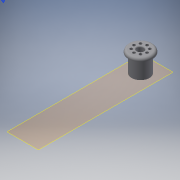
# Autodesk Inventor part: qsd
Saved by Autodesk Inventor 2018 (Build 220112000, 112)
## iProperties
Created: 2019-11-22
Part Number: qsd
Material: Generic
Document SubType Name: Modeling
Designer: bitbots
Density: 1 g/cm^3
Appearance: Default
Author: bitbots
Autodesk Inventor part; units mm, degrees
ref_plane "YZ Plane" through (0, 0, 0) normal (1, 0, 0) x (0, 1, 0)
ref_plane "XZ Plane" through (0, 0, 0) normal (0, 1, 0) x (-1, 0, 0)
ref_plane "XY Plane" through (0, 0, 0) normal (0, 0, 1) x (1, 0, 0)
ref_plane "Work Plane1" through (0, 0, 0) normal (0, 0, 1) x (1, 0, 0)
sketch "Sketch1" plane through (0, 0, 0) normal (0, 0, 1) x (1, 0, 0)
  line L0 (-11.048, 15.3384) -> (-24.0178, 163.5839) projected
  arc A0 (-11.7363, 13.6476) -> (-11.048, 15.3384) centre (-13.0404, 15.1641) ccw projected
  arc A1 (-11.7363, 13.6476) -> (9, -15.5885) centre (0, 0) ccw projected
  line L1 (13.9461, -12.7329) -> (9, -15.5885) projected
  arc A2 (13.9461, -12.7329) -> (23.8699, 6.3308) centre (3.9461, 4.5877) ccw projected
  line L2 (10.9035, 154.5385) -> (23.8699, 6.3308) projected
  arc A3 (11.6063, 156.2416) -> (10.9035, 154.5385) centre (12.8958, 154.7128) ccw projected
  arc A4 (11.6063, 156.2416) -> (-9, 185.5885) centre (0, 170) ccw projected
  line L3 (-14.0939, 182.6475) -> (-9, 185.5885) projected
  arc A5 (-14.0939, 182.6475) -> (-24.0178, 163.5839) centre (-4.0939, 165.327) ccw projected
  circle A6 centre (0, 0) radius 5.5 projected
  circle A7 centre (0, 170) radius 5.5 projected
  circle A8 centre (0, -11) radius 1.35 projected
  circle A9 centre (-7.7782, -7.7782) radius 1.35 projected
  circle A10 centre (-11, 0) radius 1.35 projected
  circle A11 centre (-7.7782, 7.7782) radius 1.35 projected
  circle A12 centre (0, 11) radius 1.35 projected
  circle A13 centre (7.7782, 7.7782) radius 1.35 projected
  circle A14 centre (11, 0) radius 1.35 projected
  circle A15 centre (7.7782, -7.7782) radius 1.35 projected
  circle A16 centre (0, 181) radius 1.35 projected
  circle A17 centre (7.7782, 177.7782) radius 1.35 projected
  circle A18 centre (11, 170) radius 1.35 projected
  circle A19 centre (7.7782, 162.2218) radius 1.35 projected
  circle A20 centre (0, 159) radius 1.35 projected
  circle A21 centre (-7.7782, 162.2218) radius 1.35 projected
  circle A22 centre (-11, 170) radius 1.35 projected
  circle A23 centre (-7.7782, 177.7782) radius 1.35 projected
  circle A24 centre (-18.943, 140) radius 1.35 projected
  circle A25 centre (9.5139, 136) radius 1.35 projected
  circle A26 centre (-16.7641, 115.0951) radius 1.35 projected
  circle A27 centre (11.6928, 111.0951) radius 1.35 projected
  circle A28 centre (-14.5852, 90.1903) radius 1.35 projected
  circle A29 centre (13.8717, 86.1903) radius 1.35 projected
  circle A30 centre (-12.4063, 65.2854) radius 1.35 projected
  circle A31 centre (16.0506, 61.2854) radius 1.35 projected
  circle A32 centre (0, 170) radius 15
  point P0 (0, 0)
  dimension "d0" = 30
  constraints: 1 centre point, 1 coincident
  measures "d0" diameter of A32
extrude "Extrusion1" add sketch "Sketch1" along normal blind 30 contours A32
sketch "Sketch2" plane through (0, 170, 30) normal (0, 0, 1) x (1, 0, 0)
  circle A0 centre (0, 0) radius 5.5 projected
  arc A1 (13.2288, -15) -> (-13.2288, -15) centre (0, 0) ccw
  circle A2 centre (0, 0) radius 5.5 construction
  circle A3 centre (-7.7782, 7.7782) radius 1.35 construction
  circle A4 centre (-11, 0) radius 1.35 construction
  circle A5 centre (-7.7782, -7.7782) radius 1.35 construction
  circle A6 centre (0, -11) radius 1.35 construction
  circle A7 centre (7.7782, -7.7782) radius 1.35 construction
  circle A8 centre (11, 0) radius 1.35 construction
  circle A9 centre (7.7782, 7.7782) radius 1.35 construction
  circle A10 centre (0, 11) radius 1.35 construction
  circle A11 centre (0, 0) radius 15 construction
  circle A12 centre (-7.7782, -7.7782) radius 1.35 projected
  circle A13 centre (-7.7782, -7.7782) radius 2.35
  circle A14 centre (0, -11) radius 2.35
  circle A15 centre (7.7782, -7.7782) radius 2.35
  circle A16 centre (11, 0) radius 1.35 projected
  circle A17 centre (11, 0) radius 2.35
  circle A18 centre (7.7782, 7.7782) radius 1.35 projected
  circle A19 centre (7.7782, 7.7782) radius 2.35
  circle A20 centre (0, 11) radius 1.35 projected
  circle A21 centre (0, 11) radius 2.35
  circle A22 centre (-7.7782, 7.7782) radius 1.35 projected
  circle A23 centre (-7.7782, 7.7782) radius 2.35
  circle A24 centre (-11, 0) radius 2.35
  circle A25 centre (0, 0) radius 5.5
  line L0 (13.2288, -15) -> (-13.2288, -15)
  point P0 (0, -170)
  dimension "d3" = 40
  dimension "d6" = 4.7
  dimension "d7" = 4.7
  dimension "d8" = 4.7
  dimension "d9" = 4.7
  dimension "d10" = 4.7
  dimension "d11" = 4.7
  dimension "d12" = 4.7
  dimension "d13" = 4.7
  constraints: 10 centre point, 10 coincident, 2 end point, 2 point on circle, 1 concentric, 1 horizontal
  measures "d3" diameter of A1
  measures "d6" diameter of A13
  measures "d7" diameter of A14
  measures "d8" diameter of A15
  measures "d9" diameter of A17
  measures "d10" diameter of A19
  measures "d11" diameter of A21
  measures "d12" diameter of A23
  measures "d13" diameter of A24
extrude "Extrusion2" add sketch "Sketch2" along normal blind 5 contours L0 A1
sketch "Sketch3" plane through (0, 159, 30) normal (0, 0, 1) x (1, 0, 0)
  line L0 (-11.048, -143.6616) -> (-24.0178, 4.5839) projected
  arc A0 (-11.7363, -145.3524) -> (-11.048, -143.6616) centre (-13.0404, -143.8359) ccw projected
  arc A1 (-11.7363, -145.3524) -> (9, -174.5885) centre (0, -159) ccw projected
  line L1 (13.9461, -171.7329) -> (9, -174.5885) projected
  arc A2 (13.9461, -171.7329) -> (23.8699, -152.6692) centre (3.9461, -154.4123) ccw projected
  line L2 (10.9035, -4.4615) -> (23.8699, -152.6692) projected
  arc A3 (11.6063, -2.7584) -> (10.9035, -4.4615) centre (12.8958, -4.2872) ccw projected
  arc A4 (11.6063, -2.7584) -> (-9, 26.5885) centre (0, 11) ccw projected
  line L3 (-14.0939, 23.6475) -> (-9, 26.5885) projected
  arc A5 (-14.0939, 23.6475) -> (-24.0178, 4.5839) centre (-4.0939, 6.327) ccw projected
  circle A6 centre (0, -159) radius 5.5 projected
  circle A7 centre (0, 11) radius 5.5 projected
  circle A8 centre (0, -170) radius 1.35 projected
  circle A9 centre (-7.7782, -166.7782) radius 1.35 projected
  circle A10 centre (-11, -159) radius 1.35 projected
  circle A11 centre (-7.7782, -151.2218) radius 1.35 projected
  circle A12 centre (0, -148) radius 1.35 projected
  circle A13 centre (7.7782, -151.2218) radius 1.35 projected
  circle A14 centre (11, -159) radius 1.35 projected
  circle A15 centre (7.7782, -166.7782) radius 1.35 projected
  circle A16 centre (0, 22) radius 1.35 projected
  circle A17 centre (7.7782, 18.7782) radius 1.35 projected
  circle A18 centre (11, 11) radius 1.35 projected
  circle A19 centre (7.7782, 3.2218) radius 1.35 projected
  circle A20 centre (0, 0) radius 1.35 projected
  circle A21 centre (-7.7782, 3.2218) radius 1.35 projected
  circle A22 centre (-11, 11) radius 1.35 projected
  circle A23 centre (-7.7782, 18.7782) radius 1.35 projected
  circle A24 centre (-18.943, -19) radius 1.35 projected
  circle A25 centre (9.5139, -23) radius 1.35 projected
  circle A26 centre (-16.7641, -43.9049) radius 1.35 projected
  circle A27 centre (11.6928, -47.9049) radius 1.35 projected
  circle A28 centre (-14.5852, -68.8097) radius 1.35 projected
  circle A29 centre (13.8717, -72.8097) radius 1.35 projected
  circle A30 centre (-12.4063, -93.7146) radius 1.35 projected
  circle A31 centre (16.0506, -97.7146) radius 1.35 projected
  circle A32 centre (0, 0) radius 2.35
  circle A33 centre (7.7782, 3.2218) radius 2.35
  circle A34 centre (11, 11) radius 2.35
  circle A35 centre (7.7782, 18.7782) radius 2.35
  circle A36 centre (0, 22) radius 2.35
  circle A37 centre (-7.7782, 18.7782) radius 2.35
  circle A38 centre (-11, 11) radius 2.35
  circle A39 centre (-7.7782, 3.2218) radius 2.35
  point P0 (0, -159)
  dimension "d15" = 4.7
  dimension "d18" = 360
  constraints: 8 centre point, 3 coincident, 23 other
  measures "d15" diameter of A32
extrude "Extrusion3" cut sketch "Sketch3" against normal blind 25 contours A32 | A33 | A34 | A35 | A36 | A37 | A38 | A39
sketch "Sketch4" plane through (7.7782, 162.2218, 5) normal (0, 0, 1) x (1, 0, 0)
  circle A0 centre (-7.7782, 7.7782) radius 5.5 projected
  circle A1 centre (-18.7782, 7.7782) radius 2.35 projected
  circle A2 centre (-15.5563, 15.5563) radius 2.35 projected
  circle A3 centre (-7.7782, 18.7782) radius 2.35 projected
  circle A4 centre (0, 15.5563) radius 2.35 projected
  circle A5 centre (3.2218, 7.7782) radius 2.35 projected
  circle A6 centre (0, 0) radius 2.35 projected
  circle A7 centre (-7.7782, -3.2218) radius 2.35 projected
  circle A8 centre (-15.5563, 0) radius 2.35 projected
  arc A9 (5.4506, -7.2218) -> (-21.0069, -7.2218) centre (-7.7782, 7.7782) ccw projected
  line L0 (-21.0069, -7.2218) -> (5.4506, -7.2218) projected
  point P0 (-7.7782, -162.2218)
extrude "Extrusion4" cut sketch "Sketch4" against normal up to next contours A2 | A4 | A6 | A8
fillet "Fillet1" radius 4 1 edges at (0, 190, 35)
fillet "Fillet2" radius 2 1 edges at (-5.5, 170, 35)
sketch "Sketch5" plane through (0, 170, 0) normal (0, 0, -1) x (-1, 0, 0)
  circle A0 centre (0, 0) radius 15 projected
  circle A1 centre (0, 0) radius 13.5
  circle A2 centre (0, 0) radius 5.5 projected
  circle A3 centre (0, 0) radius 15
  point P0 (0, -170)
  dimension "d26" = 27
  dimension "d27" = 30
  constraints: 2 centre point, 2 coincident
  measures "d26" diameter of A1
  measures "d27" diameter of A3
extrude "Extrusion5" cut sketch "Sketch5" against normal blind 30 contours A0
fillet "Fillet3" radius 1.5 5 edges at (10.2968, 155, 34.3446) (13.2288, 155, 30.5) (-10.2968, 155, 34.3446) (-13.2288, 155, 30.5) (0, 155, 35)
body "Solid1"
